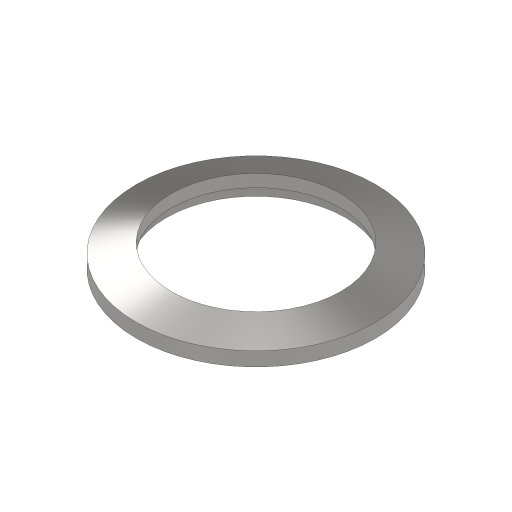
# Autodesk Inventor part: KF40_welding_part
Saved by Autodesk Inventor 2024.2 (Build 282272000, 272)
## iProperties
Created: 2022-12-02
Part Number: KF40_welding_part
Material: Stainless Steel, 440C
Document SubType Name: Modeling
Designer: kuzmin
Density: 7.75 g/cm^3
Appearance: Semi-Polished
Author: kuzmin
Autodesk Inventor part; units mm, degrees
ref_plane "YZ Plane" through (0, 0, 0) normal (1, 0, 0) x (0, 1, 0)
ref_plane "XZ Plane" through (0, 0, 0) normal (0, 1, 0) x (-1, 0, 0)
ref_plane "XY Plane" through (0, 0, 0) normal (0, 0, 1) x (1, 0, 0)
sketch "Sketch1" plane through (0, 0, 0) normal (0, 0, 1) x (1, 0, 0)
  line L0 (0, 2.5) -> (0, 6.0143)
  line L1 (0, 6.0143) -> (16.9969, 6.0143)
  line L2 (16.9969, 6.0143) -> (27.5, 3.2)
  line L3 (27.5, 3.2) -> (27.5, 0)
  line L4 (27.5, 0) -> (20.625, 0)
  line L5 (20.625, 0) -> (20.625, 2.5)
  line L6 (20.625, 2.5) -> (0, 2.5)
  line L7 (0, 0) -> (0, 22.9167)
  dimension "d0" = 55
  dimension "d1" = 3.2
  dimension "d2" = 2.5
  dimension "d3" = 41.25
  dimension "d4" = 15
  dimension "d5" = 0
  constraints: 16 end point, 3 perpendicular, 1 horizontal, 1 parallel
  measures "d0" diameter of L3 L7
  measures "d1" distance of L2.end L3.end
  measures "d2" distance of L4.end L5.end
  measures "d3" diameter of L5 L7
  measures "d4" angle of L6 L2
  measures "d5" distance between parallel lines of L0 L7
revolve "Revolution1" add sketch "Sketch1" angle 360 about axis through (0, 0, 0) along (0, 1, 0)
sketch "Sketch2" plane through (0, 6.0143, 0) normal (0, 1, 0) x (1, 0, 0)
  circle A0 centre (0, 0) radius 19.5
  dimension "d7" = 39
  constraints: 1 centre point, 1 coincident
  measures "d7" diameter of A0
extrude "Extrusion1" cut sketch "Sketch2" against normal through all
body "Solid1"
